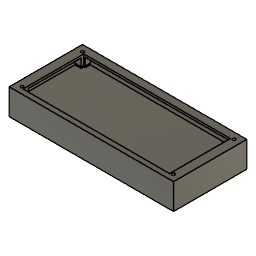
RC2004C_display_case (Autodesk Fusion 360 design; units mm, degrees)
Autodesk Fusion 360 part; units mm, degrees
note: some values were not read from the file. Set by a fixed rule: which sketch regions a step uses.
sketch "Sketch1" plane through (0, 0, 0) normal (0, 0, 1) x (1, 0, 0)
  line L0 (0, 0) -> (146, 0)
  line L1 (146, 0) -> (146, 62.5)
  line L2 (146, 62.5) -> (0, 62.5)
  line L3 (0, 62.5) -> (0, 0)
  line L4 (-0.4, -0.4) -> (146.4, -0.4)
  line L5 (146.4, -0.4) -> (146.4, 62.9)
  line L6 (146.4, 62.9) -> (-0.4, 62.9)
  line L7 (-0.4, 62.9) -> (-0.4, -0.4)
  line L8 (-2.4, -2.4) -> (148.4, -2.4)
  line L9 (148.4, -2.4) -> (148.4, 64.9)
  line L10 (148.4, 64.9) -> (-2.4, 64.9)
  line L11 (-2.4, 64.9) -> (-2.4, -2.4)
  circle A0 centre (142.5, 59) radius 1.35
  circle A1 centre (142.5, 3.5) radius 1.35
  circle A2 centre (3.5, 3.5) radius 1.35
  circle A3 centre (3.5, 59) radius 1.35
  line L12 (5.8, 57.9) -> (140.2, 57.9)
  line L13 (140.2, 57.9) -> (140.2, 2.2)
  line L14 (140.2, 2.2) -> (5.8, 2.2)
  line L15 (5.8, 2.2) -> (5.8, 57.9)
  line L16 (5.8, 7) -> (-0.4, 7)
  line L17 (7, 2.2) -> (7, -0.4)
  line L18 (5.8, 55.5) -> (-0.4, 55.5)
  line L19 (7, 57.9) -> (7, 62.9)
  line L20 (139, 57.9) -> (139, 62.9)
  line L21 (140.2, 55.5) -> (146.4, 55.5)
  line L22 (140.2, 7) -> (146.4, 7)
  line L23 (139, 2.2) -> (139, -0.4)
  point P0 (18, 60)
  dimension "d7" = 146
  dimension "d8" = 62.5
  dimension "d9" = 0.4
  dimension "d10" = 2
  dimension "d11" = 2.7
  dimension "d12" = 2.7
  dimension "d14" = 2.7
  dimension "d17" = 3.5
  dimension "d18" = 3.5
  dimension "d19" = 3.5
  dimension "d20" = 3.5
  dimension "d58" = 2.5
  dimension "d59" = 3.5
  dimension "d60" = 18
  dimension "d65" = 3.5
  dimension "d67" = 3.5
  dimension "d68" = 3.5
  dimension "d69" = 2.7
  dimension "d70" = 5.8
  dimension "d71" = 5.8
  dimension "d72" = 4.6
  dimension "d73" = 2.2
  dimension "d82" = 3.5
  dimension "d83" = 3.5
  dimension "d84" = 3.5
  dimension "d85" = 3.5
  dimension "d86" = 3.5
  dimension "d87" = 3.5
  dimension "d88" = 3.5
  dimension "d89" = 3.5
  constraint coincident L0.start L3.end
  constraint horizontal L0
  constraint vertical L1
  constraint horizontal L2
  constraint vertical L3
  constraint horizontal L12
  constraint vertical L13
  constraint horizontal L14
  constraint vertical L15
  constraint coincident L15 L16.start
  constraint coincident L7 L16.end
  constraint perpendicular L7 L16
  constraint coincident L14 L17.start
  constraint coincident L4 L17.end
  constraint perpendicular L4 L17
  constraint coincident L15 L18.start
  constraint coincident L7 L18.end
  constraint perpendicular L7 L18
  constraint coincident L12 L19.start
  constraint coincident L6 L19.end
  constraint perpendicular L6 L19
  constraint coincident L12 L20.start
  constraint coincident L6 L20.end
  constraint perpendicular L6 L20
  constraint coincident L13 L21.start
  constraint coincident L5 L21.end
  constraint perpendicular L5 L21
  constraint coincident L13 L22.start
  constraint coincident L5 L22.end
  constraint perpendicular L5 L22
  constraint coincident L14 L23.start
  constraint coincident L4 L23.end
  constraint perpendicular L4 L23
  measures "d7" distance of L1 L3
  measures "d8" distance of L0 L2
  measures "d11" diameter of A0
  measures "d12" diameter of A1
  measures "d14" diameter of A2
  measures "d17" distance of L2 A0.centre
  measures "d18" distance of L1 A0.centre
  measures "d19" distance of L1 A1.centre
  measures "d20" distance of L0 A1.centre
  measures "d58" distance of P0 L2
  measures "d59" distance of L0 A2.centre
  measures "d60" distance of P0 L3
  measures "d65" distance of L3 A2.centre
  measures "d67" distance of L2 A3.centre
  measures "d68" distance of L3 A3.centre
  measures "d69" diameter of A3
  measures "d70" distance of L3 L15
  measures "d71" distance of L1 L13
  measures "d72" distance of L2 L12
  measures "d73" distance of L0 L14
  measures "d82" distance of A1.centre L23
  measures "d83" distance of A1.centre L22
  measures "d84" distance of A0.centre L20
  measures "d85" distance of A0.centre L21
  measures "d86" distance of A3.centre L19
  measures "d87" distance of A3.centre L18
  measures "d88" distance of A2.centre L16
  measures "d89" distance of A2.centre L17
extrude "Extrude4" add sketch "Sketch1" along normal blind 9 contours L0 L3 L14 L15 L16 L17 | L0 L3 L4 L7 L16 L17 | L0 L14 L17 L23 | L0 L4 L17 L23 | L3 L7 L16 L18 | L3 L15 L16 L18 | L0 L1 L13 L14 L22 L23 | L0 L1 L4 L5 L22 L23 | L2 L3 L6 L7 L18 L19 | L2 L3 L12 L15 L18 L19 | L1 L13 L21 L22 | L1 L5 L21 L22 | L2 L6 L19 L20 | L2 L12 L19 L20 | L1 L2 L12 L13 L20 L21 | L1 L2 L5 L6 L20 L21 | L8 L9 L10 L11 makes body 1
extrude "Extrude6" cut sketch "Sketch1" along normal blind 7 contours L0 L14 L17 L23 | L0 L4 L17 L23 | L3 L7 L16 L18 | L3 L15 L16 L18 | L1 L13 L21 L22 | L1 L5 L21 L22 | L2 L6 L19 L20 | L2 L12 L19 L20 bodies 1
extrude "Extrude7" add sketch "Sketch1" against normal blind 14.8 contours L8 L9 L10 L11 bodies 1
extrude "Extrude8" add sketch "Sketch1" against normal blind 3.3 separate body contours L0 L3 L14 L15 L16 L17 | L0 L14 L17 L23 | L3 L15 L16 L18 | L0 L1 L13 L14 L22 L23 | L12 L13 L14 L15 | L2 L3 L12 L15 L18 L19 | L1 L13 L21 L22 | L2 L12 L19 L20 | L1 L2 L12 L13 L20 L21 makes body 2
extrude "Extrude9" cut sketch "Sketch1" against normal blind 1.3 contours L0 L3 L4 L7 L16 L17 | L0 L14 L17 L23 | L3 L15 L16 L18 | L0 L1 L4 L5 L22 L23 | L12 L13 L14 L15 | L2 L3 L6 L7 L18 L19 | L1 L13 L21 L22 | L2 L12 L19 L20 | L1 L2 L5 L6 L20 L21 bodies 2
sketch "Sketch3" plane through (-2.4, 0, 0) normal (-1, 0, 0) x (0, -1, 0)
  line L0 (2.4, -14.8) -> (2.4, 9)
  line L1 (2.4, 9) -> (-64.9, 9)
  line L2 (-64.9, 9) -> (-64.9, -14.8)
  line L3 (-64.9, -14.8) -> (2.4, -14.8)
  line L4 (-51, -5) -> (-38, -5)
  line L5 (-38, -5) -> (-38, -13)
  line L6 (-38, -13) -> (-51, -13)
  line L7 (-51, -13) -> (-51, -5)
  point P0 (-60, 0)
  dimension "d90" = 13
  dimension "d91" = 8
  dimension "d92" = 5
  dimension "d93" = 9
  constraint horizontal L4
  constraint vertical L5
  constraint horizontal L6
  constraint vertical L7
  measures "d90" distance of L5 L7
  measures "d91" distance of L4 L6
  measures "d92" distance of L4 origin
  measures "d93" distance of L7 P0
extrude "Extrude10" cut sketch "Sketch3" against normal blind 2 contours L4 L5 L6 L7 bodies 1
